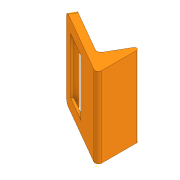
# Autodesk Inventor part: ShelfLabelStand
Saved by Autodesk Inventor 2020.3 (Build 243373000, 373)
## iProperties
Created: 2021-08-20
Part Number: ShelfLabelStand
Material: Generic
Document SubType Name: Modeling
Designer: Yusuf
Mass: 40.7468 g
Surface Area: 135.256 cm^2
Volume: 40.7468 cm^3
Density: 1 g/cm^3
Appearance: Orange
Author: Yusuf
Autodesk Inventor part; units mm, degrees
ref_plane "YZ Plane" through (0, 0, 0) normal (1, 0, 0) x (0, 1, 0)
ref_plane "XZ Plane" through (0, 0, 0) normal (0, 1, 0) x (-1, 0, 0)
ref_plane "XY Plane" through (0, 0, 0) normal (0, 0, 1) x (1, 0, 0)
sketch "Sketch1" plane through (0, 0, 0) normal (0, 1, 0) x (-1, 0, 0)
  line L0 (0, 0) -> (62.3538, -36)
  line L1 (0, 25) -> (0, -25) construction
  line L2 (62.3538, -36) -> (59.1038, -41.6292)
  line L3 (59.1038, -41.6292) -> (15.7879, -16.6207)
  line L4 (15.7879, -16.6207) -> (0, -43.9661)
  line L5 (0, 0) -> (0, -43.9661)
  dimension "d0" = 72
  dimension "d1" = 50
  dimension "d2" = 60
  dimension "d3" = 6.5
  dimension "d19" = 90
  constraints: 12 end point, 3 coincident, 2 vertical, 1 midpoint, 1 parallel
  measures "d0" distance of L0.start L0.end
  measures "d1" distance of L1.start L1.end
  measures "d2" angle of L1 L0
  measures "d3" distance of L0.end L2.end
  measures "d19" angle of L4 L3
extrude "Extrusion1" add sketch "Sketch1" along normal blind 72
sketch "Sketch2" plane through (0, 0, 0) normal (-0.5, 0, 0.8660254) x (0.8660254, 0, 0.5)
  line L0 (-62, 10.875) -> (-36.83, 10.875)
  line L1 (-36.83, 10.875) -> (-36.83, 61.125)
  line L2 (-36.83, 61.125) -> (-62, 61.125)
  line L3 (-62, 61.125) -> (-62, 10.875)
  line L4 (-72, 0) -> (-72, 72) projected
  point P0 (0, 0)
  point P1 (-62, 36)
  point P2 (-72, 36)
  dimension "d6" = 25.17
  dimension "d7" = 50.25
  dimension "d8" = 10
  constraints: 8 end point, 2 midpoint, 2 parallel, 1 horizontal, 1 horizontal alignment, 1 perpendicular
  measures "d6" distance of L2.end L1.end
  measures "d7" distance of L1.end L0.end
  measures "d8" distance between parallel lines of L3 L4
extrude "Extrusion2" cut sketch "Sketch2" against normal up to surface (6.5 mm away)
sketch "Sketch3" plane through (-59.1038, 0, -41.6292) normal (0.5, 0, -0.8660254) x (-0.8660254, 0, -0.5)
  line L0 (-6.585, 63.785) -> (-38.585, 63.785)
  line L1 (-38.585, 63.785) -> (-38.585, -1.215)
  line L2 (-38.585, -1.215) -> (-6.585, -1.215)
  line L3 (-6.585, -1.215) -> (-6.585, 63.785)
  line L4 (-35.17, 61.125) -> (-10, 61.125) projected
  point P0 (-72, 0)
  point P1 (-22.585, 63.785)
  point P2 (-22.585, 61.125)
  dimension "d11" = 32
  dimension "d12" = 65
  dimension "d13" = 2.66
  constraints: 8 end point, 2 midpoint, 2 parallel, 1 horizontal, 1 perpendicular, 1 vertical alignment
  measures "d11" distance of L2.end L1.end
  measures "d12" distance of L1.end L0.end
  measures "d13" distance between parallel lines of L4 L0
extrude "Extrusion3" cut sketch "Sketch3" against normal blind 4.5
fillet "Fillet1" radius 3 1 edges at (0, 36, 0)
fillet "Fillet2" radius 2 1 edges at (0, 36, -43.9661)
fillet "Fillet3" radius 4 2 edges at (-60.7288, 72, -38.8146) (-60.7288, 0, -38.8146)
fillet "Fillet4" radius 4 1 edges at (-15.7879, 36, -16.6207)
sketch "Sketch4" plane through (-25.6882, 0, -22.3367) normal (0.5, 0, -0.8660254) x (-0.8660254, 0, -0.5)
  circle A0 centre (35.085, 16.41) radius 1.55
  line L0 (38.585, 4) -> (38.585, 68) projected
  circle A1 centre (35.085, 47.41) radius 1.55
  circle A2 centre (-2.915, 16.41) radius 1.6
  circle A3 centre (-2.915, 47.41) radius 1.6
  point P0 (-33.415, 0)
  point P1 (34.585, 0)
  dimension "d21" = 3.1
  dimension "d22" = 16.41
  dimension "d23" = 3.5
  dimension "d24" = 3.1
  dimension "d25" = 31
  dimension "d26" = 3.2
  dimension "d27" = 38
  dimension "d28" = 3.2
  dimension "d29" = 38
  constraints: 4 centre point, 2 vertical alignment, 1 horizontal alignment
  measures "d21" diameter of A0
  measures "d22" vertical distance of A0.centre point (34.585, 0)
  measures "d23" distance from line of A0.centre L0
  measures "d24" diameter of A1
  measures "d25" distance of A0.centre A1.centre
  measures "d26" diameter of A2
  measures "d27" distance of A2.centre A0.centre
  measures "d28" diameter of A3
  measures "d29" distance of A3.centre A1.centre
extrude "Extrusion4" cut sketch "Sketch4" against normal up to surface (4.5 mm away)
sketch "Sketch5" plane through (0, 0, 0) normal (0, -1, 0) x (1, 0, 0)
  line L0 (-11.1256, -19.2586) -> (-11.1256, -9.2074) construction
  line L1 (-11.1256, -9.2074) -> (-1.0319, -9.2074) construction
  line L2 (-1.0319, -9.2074) -> (-1.0319, -19.2586) construction
  line L3 (-1.0319, -19.2586) -> (-11.1256, -19.2586) construction
  arc A0 (-8.7423, -17.7336) -> (-8.7372, -10.7469) centre (-6.0502, -14.2422) ccw
  arc A1 (-9.1232, -18.214) -> (-9.1477, -10.2896) centre (-6.0502, -14.2422) ccw
  arc A2 (-9.1477, -10.2896) -> (-8.7372, -10.7469) centre (-8.8163, -10.405) ccw
  arc A3 (-8.7423, -17.7336) -> (-9.1232, -18.214) centre (-8.8713, -18.0225) ccw
  line L4 (-4.6557, -14.5422) -> (-7.2177, -14.5422)
  line L5 (-7.2177, -14.5422) -> (-7.2177, -13.9533)
  line L6 (-7.2177, -13.9533) -> (-4.6557, -13.9533)
  line L7 (-4.6557, -13.9533) -> (-4.6557, -14.5422)
  arc A4 (-4.6557, -14.5422) -> (-4.6557, -13.9533) centre (-4.7199, -14.2478) ccw
  arc A5 (-7.2177, -13.9533) -> (-7.2177, -14.5422) centre (-7.171, -14.2478) ccw
  arc A6 (-8.2247, -12.6322) -> (-8.1705, -15.9511) centre (-6.0663, -14.2568) ccw
  arc A7 (-7.7175, -12.932) -> (-7.6745, -15.6001) centre (-6.057, -14.2396) ccw
  arc A8 (-8.6126, -12.2607) -> (-8.5782, -16.3059) centre (-6.0095, -14.2613) ccw
  arc A9 (-9.1192, -11.9337) -> (-9.0775, -16.6329) centre (-6.1136, -14.2568) ccw
  arc A10 (-9.5852, -11.4861) -> (-9.568, -17.0116) centre (-5.9362, -14.2375) ccw
  point P0 (0, 0)
  constraints: 22 point on circle, 11 centre point, 8 end point, 3 perpendicular, 1 coincident, 1 horizontal, 2 other
body "Solid1"
